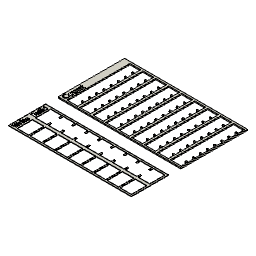
magnetic math (Autodesk Fusion 360 design; units mm, degrees)
Autodesk Fusion 360 part; units mm, degrees
sketch "Sketch3" plane through (0, 0, 0) normal (0, 0, 1) x (1, 0, 0)
  line L0 (672.1477, -0.2754) -> (0.2647, -0.2754)
  line L1 (0.2647, -0.2754) -> (0.2647, -203.3998)
  line L2 (0.2647, -203.3998) -> (672.1477, -203.3998)
  line L3 (672.1477, -203.3998) -> (672.1477, -0.2754)
  line L4 (100.5154, -109.9886) -> (37.7823, -109.9886)
  line L5 (37.7823, -109.9886) -> (37.7823, -193.6499)
  line L6 (37.7823, -193.6499) -> (100.5154, -193.6499)
  line L7 (100.5154, -193.6499) -> (100.5154, -109.9886)
  line L8 (170.7886, -109.9886) -> (108.056, -109.9886)
  line L9 (108.056, -109.9886) -> (108.056, -193.6499)
  line L10 (108.056, -193.6499) -> (170.7886, -193.6499)
  line L11 (170.7886, -193.6499) -> (170.7886, -109.9886)
  line L12 (241.0619, -109.9886) -> (178.3293, -109.9886)
  line L13 (178.3293, -109.9886) -> (178.3293, -193.6499)
  line L14 (178.3293, -193.6499) -> (241.0619, -193.6499)
  line L15 (241.0619, -193.6499) -> (241.0619, -109.9886)
  line L16 (311.3615, -109.9886) -> (248.6025, -109.9886)
  line L17 (248.6025, -109.9886) -> (248.6025, -193.6499)
  line L18 (248.6025, -193.6499) -> (311.3615, -193.6499)
  line L19 (311.3615, -193.6499) -> (311.3615, -109.9886)
  line L20 (381.6352, -109.9886) -> (318.8757, -109.9886)
  line L21 (318.8757, -109.9886) -> (318.8757, -193.6499)
  line L22 (318.8757, -193.6499) -> (381.6352, -193.6499)
  line L23 (381.6352, -193.6499) -> (381.6352, -109.9886)
  line L24 (451.9084, -109.9886) -> (389.149, -109.9886)
  line L25 (389.149, -109.9886) -> (389.149, -193.6499)
  line L26 (389.149, -193.6499) -> (451.9084, -193.6499)
  line L27 (451.9084, -193.6499) -> (451.9084, -109.9886)
  line L28 (522.1817, -109.9886) -> (459.4491, -109.9886)
  line L29 (459.4491, -109.9886) -> (459.4491, -193.6499)
  line L30 (459.4491, -193.6499) -> (522.1817, -193.6499)
  line L31 (522.1817, -193.6499) -> (522.1817, -109.9886)
  line L32 (592.4549, -109.9886) -> (529.7223, -109.9886)
  line L33 (529.7223, -109.9886) -> (529.7223, -193.6499)
  line L34 (529.7223, -193.6499) -> (592.4549, -193.6499)
  line L35 (592.4549, -193.6499) -> (592.4549, -109.9886)
  line L36 (662.7281, -109.9886) -> (599.9955, -109.9886)
  line L37 (599.9955, -109.9886) -> (599.9955, -193.6499)
  line L38 (599.9955, -193.6499) -> (662.7281, -193.6499)
  line L39 (662.7281, -193.6499) -> (662.7281, -109.9886)
  line L40 (100.5154, -28.7041) -> (100.5154, -10.038)
  line L41 (100.5154, -10.038) -> (37.7823, -10.038)
  line L42 (37.7823, -10.038) -> (37.7823, -93.6982)
  line L43 (37.7823, -93.6982) -> (100.5154, -93.6982)
  line L44 (100.5154, -93.6982) -> (100.5154, -75.5793)
  line L45 (100.5154, -75.5793) -> (108.056, -75.5793)
  line L46 (108.056, -75.5793) -> (108.056, -93.6982)
  line L47 (108.056, -93.6982) -> (170.7886, -93.6982)
  line L48 (170.7886, -93.6982) -> (170.7886, -75.5793)
  line L49 (170.7886, -75.5793) -> (178.3293, -75.5793)
  line L50 (178.3293, -75.5793) -> (178.3293, -93.6982)
  line L51 (178.3293, -93.6982) -> (241.0619, -93.6982)
  line L52 (241.0619, -93.6982) -> (241.0619, -75.5793)
  line L53 (241.0619, -75.5793) -> (248.6025, -75.5793)
  line L54 (248.6025, -75.5793) -> (248.6025, -93.6982)
  line L55 (248.6025, -93.6982) -> (311.3615, -93.6982)
  line L56 (311.3615, -93.6982) -> (311.3615, -75.5793)
  line L57 (311.3615, -75.5793) -> (318.8757, -75.5793)
  line L58 (318.8757, -75.5793) -> (318.8757, -93.6982)
  line L59 (318.8757, -93.6982) -> (381.6352, -93.6982)
  line L60 (381.6352, -93.6982) -> (381.6352, -75.5793)
  line L61 (381.6352, -75.5793) -> (389.149, -75.5793)
  line L62 (389.149, -75.5793) -> (389.149, -93.6982)
  line L63 (389.149, -93.6982) -> (451.9084, -93.6982)
  line L64 (451.9084, -93.6982) -> (451.9084, -75.5793)
  line L65 (451.9084, -75.5793) -> (459.4491, -75.5793)
  line L66 (459.4491, -75.5793) -> (459.4491, -93.6982)
  line L67 (459.4491, -93.6982) -> (522.1817, -93.6982)
  line L68 (522.1817, -93.6982) -> (522.1817, -75.5793)
  line L69 (522.1817, -75.5793) -> (529.7223, -75.5793)
  line L70 (529.7223, -75.5793) -> (529.7223, -93.6982)
  line L71 (529.7223, -93.6982) -> (592.4549, -93.6982)
  line L72 (592.4549, -93.6982) -> (592.4549, -75.5793)
  line L73 (592.4549, -75.5793) -> (599.9955, -75.5793)
  line L74 (599.9955, -75.5793) -> (599.9955, -93.6982)
  line L75 (599.9955, -93.6982) -> (662.7281, -93.6982)
  line L76 (662.7281, -93.6982) -> (662.7281, -10.038)
  line L77 (662.7281, -10.038) -> (599.9955, -10.038)
  line L78 (599.9955, -10.038) -> (599.9955, -28.7041)
  line L79 (599.9955, -28.7041) -> (592.4549, -28.7041)
  line L80 (592.4549, -28.7041) -> (592.4549, -10.038)
  line L81 (592.4549, -10.038) -> (529.7223, -10.038)
  line L82 (529.7223, -10.038) -> (529.7223, -28.7041)
  line L83 (529.7223, -28.7041) -> (522.1817, -28.7041)
  line L84 (522.1817, -28.7041) -> (522.1817, -10.038)
  line L85 (522.1817, -10.038) -> (459.4491, -10.038)
  line L86 (459.4491, -10.038) -> (459.4491, -28.7041)
  line L87 (459.4491, -28.7041) -> (451.9084, -28.7041)
  line L88 (451.9084, -28.7041) -> (451.9084, -10.038)
  line L89 (451.9084, -10.038) -> (389.149, -10.038)
  line L90 (389.149, -10.038) -> (389.149, -28.7041)
  line L91 (389.149, -28.7041) -> (381.6352, -28.7041)
  line L92 (381.6352, -28.7041) -> (381.6352, -10.038)
  line L93 (381.6352, -10.038) -> (318.8757, -10.038)
  line L94 (318.8757, -10.038) -> (318.8757, -28.7041)
  line L95 (318.8757, -28.7041) -> (311.3615, -28.7041)
  line L96 (311.3615, -28.7041) -> (311.3615, -10.038)
  line L97 (311.3615, -10.038) -> (248.6025, -10.038)
  line L98 (248.6025, -10.038) -> (248.6025, -28.7041)
  line L99 (248.6025, -28.7041) -> (241.0619, -28.7041)
  line L100 (241.0619, -28.7041) -> (241.0619, -10.038)
  line L101 (241.0619, -10.038) -> (178.3293, -10.038)
  line L102 (178.3293, -10.038) -> (178.3293, -28.7041)
  line L103 (178.3293, -28.7041) -> (170.7886, -28.7041)
  line L104 (170.7886, -28.7041) -> (170.7886, -10.038)
  line L105 (170.7886, -10.038) -> (108.056, -10.038)
  line L106 (108.056, -10.038) -> (108.056, -28.7041)
  line L107 (108.056, -28.7041) -> (100.5154, -28.7041)
  line L108 (28.8958, -89.0962) -> (7.0937, -89.0962)
  line L109 (7.0937, -89.0962) -> (7.0937, -81.6748)
  spline S0 degree 3 poles (7.0937, -81.6748) (7.0937, -79.4876) (7.5059, -77.821) (8.3302, -76.6751) knots 0 0 0 0 1 1 1 1
  spline S1 degree 3 poles (8.3302, -76.6751) (9.1562, -75.5295) (10.3585, -74.9695) (11.9405, -74.9695) knots 0 0 0 0 1 1 1 1
  spline S2 degree 3 poles (11.9405, -74.9695) (14.5623, -74.9695) (16.4179, -76.7013) (17.5091, -80.1905) knots 0 0 0 0 1 1 1 1
  spline S3 degree 3 poles (17.5091, -80.1905) (18.501, -76.1154) (20.4986, -74.0843) (23.5034, -74.0843) knots 0 0 0 0 1 1 1 1
  spline S4 degree 3 poles (23.5034, -74.0843) (25.2428, -74.0843) (26.575, -74.6702) (27.5037, -75.868) knots 0 0 0 0 1 1 1 1
  spline S5 degree 3 poles (27.5037, -75.868) (28.4324, -77.0657) (28.8958, -78.7715) (28.8958, -80.9979) knots 0 0 0 0 1 1 1 1
  line L110 (28.8958, -80.9979) -> (28.8958, -89.0962)
  line L111 (16.1682, -84.8126) -> (16.1682, -83.7451)
  spline S6 degree 3 poles (16.1682, -83.7451) (16.1682, -82.469) (15.8535, -81.4536) (15.2259, -80.6983) knots 0 0 0 0 1 1 1 1
  spline S7 degree 3 poles (15.2259, -80.6983) (14.5965, -79.9563) (13.7414, -79.5787) (12.6622, -79.5787) knots 0 0 0 0 1 1 1 1
  spline S8 degree 3 poles (12.6622, -79.5787) (11.66, -79.5787) (10.9793, -79.8782) (10.6219, -80.4771) knots 0 0 0 0 1 1 1 1
  spline S9 degree 3 poles (10.6219, -80.4771) (10.2628, -81.0889) (10.0832, -82.2218) (10.0832, -83.9012) knots 0 0 0 0 1 1 1 1
  line L112 (10.0832, -83.9012) -> (10.0832, -84.8126)
  line L113 (10.0832, -84.8126) -> (16.1682, -84.8126)
  line L114 (25.802, -84.8126) -> (25.802, -83.8493)
  spline S10 degree 3 poles (25.802, -83.8493) (25.802, -81.9352) (25.5985, -80.6332) (25.1914, -79.9042) knots 0 0 0 0 1 1 1 1
  spline S11 degree 3 poles (25.1914, -79.9042) (24.7827, -79.1881) (24.0405, -78.8234) (22.9596, -78.8234) knots 0 0 0 0 1 1 1 1
  spline S12 degree 3 poles (22.9596, -78.8234) (21.8496, -78.8234) (20.9261, -79.3053) (20.189, -80.2688) knots 0 0 0 0 1 1 1 1
  spline S13 degree 3 poles (20.189, -80.2688) (19.4536, -81.2453) (19.0842, -82.456) (19.0842, -83.9404) knots 0 0 0 0 1 1 1 1
  line L115 (19.0842, -83.9404) -> (19.0842, -84.8126)
  line L116 (19.0842, -84.8126) -> (25.802, -84.8126)
  line L117 (28.8958, -60.0879) -> (25.8465, -60.0879)
  spline S14 degree 3 poles (25.8465, -60.0879) (28.1245, -61.4939) (29.2635, -63.3296) (29.2635, -65.5952) knots 0 0 0 0 1 1 1 1
  spline S15 degree 3 poles (29.2635, -65.5952) (29.2635, -67.0403) (28.8086, -68.1732) (27.8936, -69.0065) knots 0 0 0 0 1 1 1 1
  spline S16 degree 3 poles (27.8936, -69.0065) (26.9804, -69.8528) (25.7336, -70.2694) (24.1533, -70.2694) knots 0 0 0 0 1 1 1 1
  line L118 (24.1533, -70.2694) -> (12.7204, -70.2694)
  line L119 (12.7204, -70.2694) -> (12.7204, -65.9077)
  line L120 (12.7204, -65.9077) -> (23.0776, -65.9077)
  spline S17 degree 3 poles (23.0776, -65.9077) (24.9144, -65.9077) (25.8328, -65.2958) (25.8328, -64.0589) knots 0 0 0 0 1 1 1 1
  spline S18 degree 3 poles (25.8328, -64.0589) (25.8328, -62.6918) (24.8545, -61.3637) (22.8997, -60.0879) knots 0 0 0 0 1 1 1 1
  line L121 (22.8997, -60.0879) -> (12.7204, -60.0879)
  line L122 (12.7204, -60.0879) -> (12.7204, -55.7262)
  line L123 (12.7204, -55.7262) -> (28.8958, -55.7262)
  line L124 (28.8958, -55.7262) -> (28.8958, -60.0879)
  line L125 (28.8958, -50.2707) -> (12.7204, -50.2707)
  line L126 (12.7204, -50.2707) -> (12.7204, -45.909)
  line L127 (12.7204, -45.909) -> (28.8958, -45.909)
  line L128 (28.8958, -45.909) -> (28.8958, -50.2707)
  line L129 (9.996, -50.2707) -> (6.3566, -50.2707)
  line L130 (6.3566, -50.2707) -> (6.3566, -45.909)
  line L131 (6.3566, -45.909) -> (9.996, -45.909)
  line L132 (9.996, -45.909) -> (9.996, -50.2707)
  line L133 (5.6349, -40.4666) -> (5.6349, -36.106)
  line L134 (5.6349, -36.106) -> (28.8965, -36.106)
  line L135 (28.8965, -36.106) -> (28.8965, -40.4666)
  line L136 (28.8965, -40.4666) -> (5.6349, -40.4666)
  line L137 (28.8958, -20.4679) -> (25.8465, -20.4679)
  spline S19 degree 3 poles (25.8465, -20.4679) (28.1245, -21.5876) (29.2635, -23.3583) (29.2635, -25.754) knots 0 0 0 0 1 1 1 1
  spline S20 degree 3 poles (29.2635, -25.754) (29.2635, -27.707) (28.5521, -29.2305) (27.1274, -30.3372) knots 0 0 0 0 1 1 1 1
  spline S21 degree 3 poles (27.1274, -30.3372) (25.7045, -31.4568) (23.7446, -32.0036) (21.2511, -32.0036) knots 0 0 0 0 1 1 1 1
  spline S22 degree 3 poles (21.2511, -32.0036) (18.5403, -32.0036) (16.3786, -31.3788) (14.7675, -30.1287) knots 0 0 0 0 1 1 1 1
  spline S23 degree 3 poles (14.7675, -30.1287) (13.1582, -28.8788) (12.3527, -27.1992) (12.3527, -25.0771) knots 0 0 0 0 1 1 1 1
  spline S24 degree 3 poles (12.3527, -25.0771) (12.3527, -23.3974) (13.0197, -21.861) (14.3554, -20.4679) knots 0 0 0 0 1 1 1 1
  line L138 (14.3554, -20.4679) -> (5.6348, -20.4679)
  line L139 (5.6348, -20.4679) -> (5.6348, -16.0933)
  line L140 (5.6348, -16.0933) -> (28.8958, -16.0933)
  line L141 (28.8958, -16.0933) -> (28.8958, -20.4679)
  spline S25 degree 3 poles (16.9481, -20.4679) (15.7697, -21.5225) (15.1814, -22.6422) (15.1814, -23.8402) knots 0 0 0 0 1 1 1 1
  spline S26 degree 3 poles (15.1814, -23.8402) (15.1814, -24.9207) (15.6962, -25.767) (16.7275, -26.405) knots 0 0 0 0 1 1 1 1
  spline S27 degree 3 poles (16.7275, -26.405) (17.7587, -27.043) (19.144, -27.3685) (20.8816, -27.3685) knots 0 0 0 0 1 1 1 1
  spline S28 degree 3 poles (20.8816, -27.3685) (24.1927, -27.3685) (25.8465, -26.301) (25.8465, -24.1786) knots 0 0 0 0 1 1 1 1
  spline S29 degree 3 poles (25.8465, -24.1786) (25.8465, -22.8896) (25.017, -21.6527) (23.3564, -20.4679) knots 0 0 0 0 1 1 1 1
  line L142 (23.3564, -20.4679) -> (16.9481, -20.4679)
  line L143 (28.8958, -187.9119) -> (7.0937, -193.3379)
  line L144 (7.0937, -193.3379) -> (7.0937, -189.0572)
  line L145 (7.0937, -189.0572) -> (23.0485, -185.0761)
  line L146 (23.0485, -185.0761) -> (7.0937, -181.3269)
  line L147 (7.0937, -181.3269) -> (7.0937, -177.5369)
  line L148 (7.0937, -177.5369) -> (22.9596, -173.9648)
  line L149 (22.9596, -173.9648) -> (7.0937, -169.7794)
  line L150 (7.0937, -169.7794) -> (7.0937, -166.6437)
  line L151 (7.0937, -166.6437) -> (28.8958, -172.3698)
  line L152 (28.8958, -172.3698) -> (28.8958, -176.6915)
  line L153 (28.8958, -176.6915) -> (13.9432, -180.0591)
  line L154 (13.9432, -180.0591) -> (28.8958, -183.5764)
  line L155 (28.8958, -183.5764) -> (28.8958, -187.9119)
  line L156 (28.8958, -163.6579) -> (12.7204, -163.6579)
  line L157 (12.7204, -163.6579) -> (12.7204, -159.2952)
  line L158 (12.7204, -159.2952) -> (15.7697, -159.2952)
  spline S30 degree 3 poles (15.7697, -159.2952) (13.4917, -158.1635) (12.3527, -156.4458) (12.3527, -154.1417) knots 0 0 0 0 1 1 1 1
  spline S31 degree 3 poles (12.3527, -154.1417) (12.3527, -153.869) (12.3818, -153.5963) (12.4399, -153.3237) knots 0 0 0 0 1 1 1 1
  line L159 (12.4399, -153.3237) -> (16.3307, -153.3237)
  spline S32 degree 3 poles (16.3307, -153.3237) (16.1032, -153.951) (15.9904, -154.5235) (15.9904, -155.0553) knots 0 0 0 0 1 1 1 1
  spline S33 degree 3 poles (15.9904, -155.0553) (15.9904, -156.7866) (16.8694, -158.2045) (18.6275, -159.2952) knots 0 0 0 0 1 1 1 1
  line L160 (18.6275, -159.2952) -> (28.8958, -159.2952)
  line L161 (28.8958, -159.2952) -> (28.8958, -163.6579)
  line L162 (28.8958, -149.9427) -> (12.7204, -149.9427)
  line L163 (12.7204, -149.9427) -> (12.7204, -145.58)
  line L164 (12.7204, -145.58) -> (28.8958, -145.58)
  line L165 (28.8958, -145.58) -> (28.8958, -149.9427)
  line L166 (9.996, -149.9427) -> (6.3566, -149.9427)
  line L167 (6.3566, -149.9427) -> (6.3566, -145.58)
  line L168 (6.3566, -145.58) -> (9.996, -145.58)
  line L169 (9.996, -145.58) -> (9.996, -149.9427)
  spline S34 degree 3 poles (28.8086, -131.7966) (29.113, -132.8327) (29.2635, -133.6507) (29.2635, -134.2506) knots 0 0 0 0 1 1 1 1
  spline S35 degree 3 poles (29.2635, -134.2506) (29.2635, -138.027) (27.4969, -139.9221) (23.9601, -139.9221) knots 0 0 0 0 1 1 1 1
  line L170 (23.9601, -139.9221) -> (15.4465, -139.9221)
  line L171 (15.4465, -139.9221) -> (15.4465, -141.7352)
  line L172 (15.4465, -141.7352) -> (12.7204, -141.7352)
  line L173 (12.7204, -141.7352) -> (12.7204, -139.9221)
  line L174 (12.7204, -139.9221) -> (9.996, -139.9221)
  line L175 (9.996, -139.9221) -> (9.4949, -135.5594)
  line L176 (9.4949, -135.5594) -> (12.7204, -135.5594)
  line L177 (12.7204, -135.5594) -> (12.7204, -132.0964)
  line L178 (12.7204, -132.0964) -> (15.4465, -132.0964)
  line L179 (15.4465, -132.0964) -> (15.4465, -135.5594)
  line L180 (15.4465, -135.5594) -> (23.3872, -135.5594)
  spline S36 degree 3 poles (23.3872, -135.5594) (25.371, -135.5594) (26.363, -134.755) (26.363, -133.1325) knots 0 0 0 0 1 1 1 1
  spline S37 degree 3 poles (26.363, -133.1325) (26.363, -132.7645) (26.2928, -132.3145) (26.156, -131.7966) knots 0 0 0 0 1 1 1 1
  line L181 (26.156, -131.7966) -> (28.8086, -131.7966)
  spline S38 degree 3 poles (28.352, -114.7273) (28.9608, -116.7998) (29.2635, -118.7628) (29.2635, -120.6307) knots 0 0 0 0 1 1 1 1
  spline S39 degree 3 poles (29.2635, -120.6307) (29.2635, -123.33) (28.4991, -125.457) (26.9667, -127.0249) knots 0 0 0 0 1 1 1 1
  spline S40 degree 3 poles (26.9667, -127.0249) (25.4343, -128.5789) (23.3427, -129.3562) (20.6901, -129.3562) knots 0 0 0 0 1 1 1 1
  spline S41 degree 3 poles (20.6901, -129.3562) (18.1863, -129.3562) (16.1699, -128.6471) (14.6427, -127.2156) knots 0 0 0 0 1 1 1 1
  spline S42 degree 3 poles (14.6427, -127.2156) (13.1154, -125.784) (12.3527, -123.9028) (12.3527, -121.5577) knots 0 0 0 0 1 1 1 1
  spline S43 degree 3 poles (12.3527, -121.5577) (12.3527, -119.1856) (13.0983, -117.454) (14.5914, -116.3634) knots 0 0 0 0 1 1 1 1
  spline S44 degree 3 poles (14.5914, -116.3634) (16.0844, -115.2727) (18.4463, -114.7273) (21.6769, -114.7273) knots 0 0 0 0 1 1 1 1
  line L182 (21.6769, -114.7273) -> (21.6769, -124.7615)
  spline S45 degree 3 poles (21.6769, -124.7615) (24.7622, -124.4753) (26.3031, -122.7711) (26.3031, -119.6764) knots 0 0 0 0 1 1 1 1
  spline S46 degree 3 poles (26.3031, -119.6764) (26.3031, -118.2175) (25.9645, -116.5679) (25.2872, -114.7273) knots 0 0 0 0 1 1 1 1
  line L183 (25.2872, -114.7273) -> (28.352, -114.7273)
  line L184 (19.2176, -124.8297) -> (19.2176, -119.0219)
  spline S47 degree 3 poles (19.2176, -119.0219) (16.4573, -119.0219) (15.0771, -119.9081) (15.0771, -121.6804) knots 0 0 0 0 1 1 1 1
  spline S48 degree 3 poles (15.0771, -121.6804) (15.0771, -123.4938) (16.4573, -124.5434) (19.2176, -124.8297) knots 0 0 0 0 1 1 1 1
extrude "Extrude3" add sketch "Sketch3" along normal blind 2 contours L0 L1 L2 L3 makes body 1
scale "Scale3" factor 0.32 about (0.2647, -203.3998, 2) bodies 1
sketch "Sketch5" plane through (0, 0, 0) normal (0, 0, 1) x (1, 0, 0)
  line L0 (215.0872, -0.0882) -> (0.0847, -0.0882)
  line L1 (0.0847, -0.0882) -> (0.0847, -116.5435)
  line L2 (0.0847, -116.5435) -> (215.0872, -116.5435)
  line L3 (215.0872, -116.5435) -> (215.0872, -0.0882)
  line L4 (27.5336, -13.7736) -> (31.5892, -13.7736)
  line L5 (31.5892, -13.7736) -> (31.5892, -3.2736)
  line L6 (31.5892, -3.2736) -> (12.5899, -3.2736)
  line L7 (12.5899, -3.2736) -> (12.5899, -7.2379)
  line L8 (12.5899, -7.2379) -> (12.5307, -7.2379)
  line L9 (12.5307, -7.2379) -> (12.5307, -109.3934)
  line L10 (12.5307, -109.3934) -> (12.5899, -109.3934)
  line L11 (12.5899, -109.3934) -> (12.5899, -113.7732)
  line L12 (12.5899, -113.7732) -> (31.5892, -113.7732)
  line L13 (31.5892, -113.7732) -> (31.5892, -103.2737)
  line L14 (31.5892, -103.2737) -> (27.5336, -103.2737)
  line L15 (27.5336, -103.2737) -> (27.5336, -101.2739)
  line L16 (27.5336, -101.2739) -> (31.5892, -101.2739)
  line L17 (31.5892, -101.2739) -> (31.5892, -90.7735)
  line L18 (31.5892, -90.7735) -> (27.5336, -90.7735)
  line L19 (27.5336, -90.7735) -> (27.5336, -88.7737)
  line L20 (27.5336, -88.7737) -> (31.5892, -88.7737)
  line L21 (31.5892, -88.7737) -> (31.5892, -78.2733)
  line L22 (31.5892, -78.2733) -> (27.5336, -78.2733)
  line L23 (27.5336, -78.2733) -> (27.5336, -76.2735)
  line L24 (27.5336, -76.2735) -> (31.5892, -76.2735)
  line L25 (31.5892, -76.2735) -> (31.5892, -65.774)
  line L26 (31.5892, -65.774) -> (27.5336, -65.774)
  line L27 (27.5336, -65.774) -> (27.5336, -63.7733)
  line L28 (27.5336, -63.7733) -> (31.5892, -63.7733)
  line L29 (31.5892, -63.7733) -> (31.5892, -53.2738)
  line L30 (31.5892, -53.2738) -> (27.5336, -53.2738)
  line L31 (27.5336, -53.2738) -> (27.5336, -51.274)
  line L32 (27.5336, -51.274) -> (31.5892, -51.274)
  line L33 (31.5892, -51.274) -> (31.5892, -40.7736)
  line L34 (31.5892, -40.7736) -> (27.5336, -40.7736)
  line L35 (27.5336, -40.7736) -> (27.5336, -38.7738)
  line L36 (27.5336, -38.7738) -> (31.5892, -38.7738)
  line L37 (31.5892, -38.7738) -> (31.5892, -28.2734)
  line L38 (31.5892, -28.2734) -> (27.5336, -28.2734)
  line L39 (27.5336, -28.2734) -> (27.5336, -26.2735)
  line L40 (27.5336, -26.2735) -> (31.5892, -26.2735)
  line L41 (31.5892, -26.2735) -> (31.5892, -15.7736)
  line L42 (31.5892, -15.7736) -> (27.5336, -15.7736)
  line L43 (27.5336, -15.7736) -> (27.5336, -13.7736)
  line L44 (50.2073, -13.7736) -> (54.2713, -13.7736)
  line L45 (54.2713, -13.7736) -> (54.2713, -3.2736)
  line L46 (54.2713, -3.2736) -> (35.2722, -3.2736)
  line L47 (35.2722, -3.2736) -> (35.2722, -7.2379)
  line L48 (35.2722, -7.2379) -> (35.2044, -7.2379)
  line L49 (35.2044, -7.2379) -> (35.2044, -109.3934)
  line L50 (35.2044, -109.3934) -> (35.2722, -109.3934)
  line L51 (35.2722, -109.3934) -> (35.2722, -113.7732)
  line L52 (35.2722, -113.7732) -> (54.2713, -113.7732)
  line L53 (54.2713, -113.7732) -> (54.2713, -103.2737)
  line L54 (54.2713, -103.2737) -> (50.2073, -103.2737)
  line L55 (50.2073, -103.2737) -> (50.2073, -101.2739)
  line L56 (50.2073, -101.2739) -> (54.2713, -101.2739)
  line L57 (54.2713, -101.2739) -> (54.2713, -90.7735)
  line L58 (54.2713, -90.7735) -> (50.2073, -90.7735)
  line L59 (50.2073, -90.7735) -> (50.2073, -88.7737)
  line L60 (50.2073, -88.7737) -> (54.2713, -88.7737)
  line L61 (54.2713, -88.7737) -> (54.2713, -78.2733)
  line L62 (54.2713, -78.2733) -> (50.2073, -78.2733)
  line L63 (50.2073, -78.2733) -> (50.2073, -76.2735)
  line L64 (50.2073, -76.2735) -> (54.2713, -76.2735)
  line L65 (54.2713, -76.2735) -> (54.2713, -65.774)
  line L66 (54.2713, -65.774) -> (50.2073, -65.774)
  line L67 (50.2073, -65.774) -> (50.2073, -63.7733)
  line L68 (50.2073, -63.7733) -> (54.2713, -63.7733)
  line L69 (54.2713, -63.7733) -> (54.2713, -53.2738)
  line L70 (54.2713, -53.2738) -> (50.2073, -53.2738)
  line L71 (50.2073, -53.2738) -> (50.2073, -51.274)
  line L72 (50.2073, -51.274) -> (54.2713, -51.274)
  line L73 (54.2713, -51.274) -> (54.2713, -40.7736)
  line L74 (54.2713, -40.7736) -> (50.2073, -40.7736)
  line L75 (50.2073, -40.7736) -> (50.2073, -38.7738)
  line L76 (50.2073, -38.7738) -> (54.2713, -38.7738)
  line L77 (54.2713, -38.7738) -> (54.2713, -28.2734)
  line L78 (54.2713, -28.2734) -> (50.2073, -28.2734)
  line L79 (50.2073, -28.2734) -> (50.2073, -26.2735)
  line L80 (50.2073, -26.2735) -> (54.2713, -26.2735)
  line L81 (54.2713, -26.2735) -> (54.2713, -15.7736)
  line L82 (54.2713, -15.7736) -> (50.2073, -15.7736)
  line L83 (50.2073, -15.7736) -> (50.2073, -13.7736)
  line L84 (72.881, -13.7736) -> (76.945, -13.7736)
  line L85 (76.945, -13.7736) -> (76.945, -3.2736)
  line L86 (76.945, -3.2736) -> (57.9459, -3.2736)
  line L87 (57.9459, -3.2736) -> (57.9459, -7.2379)
  line L88 (57.9459, -7.2379) -> (57.8782, -7.2379)
  line L89 (57.8782, -7.2379) -> (57.8782, -109.3934)
  line L90 (57.8782, -109.3934) -> (57.9459, -109.3934)
  line L91 (57.9459, -109.3934) -> (57.9459, -113.7732)
  line L92 (57.9459, -113.7732) -> (76.945, -113.7732)
  line L93 (76.945, -113.7732) -> (76.945, -103.2737)
  line L94 (76.945, -103.2737) -> (72.881, -103.2737)
  line L95 (72.881, -103.2737) -> (72.881, -101.2739)
  line L96 (72.881, -101.2739) -> (76.945, -101.2739)
  line L97 (76.945, -101.2739) -> (76.945, -90.7735)
  line L98 (76.945, -90.7735) -> (72.881, -90.7735)
  line L99 (72.881, -90.7735) -> (72.881, -88.7737)
  line L100 (72.881, -88.7737) -> (76.945, -88.7737)
  line L101 (76.945, -88.7737) -> (76.945, -78.2733)
  line L102 (76.945, -78.2733) -> (72.881, -78.2733)
  line L103 (72.881, -78.2733) -> (72.881, -76.2735)
  line L104 (72.881, -76.2735) -> (76.945, -76.2735)
  line L105 (76.945, -76.2735) -> (76.945, -65.774)
  line L106 (76.945, -65.774) -> (72.881, -65.774)
  line L107 (72.881, -65.774) -> (72.881, -63.7733)
  line L108 (72.881, -63.7733) -> (76.945, -63.7733)
  line L109 (76.945, -63.7733) -> (76.945, -53.2738)
  line L110 (76.945, -53.2738) -> (72.881, -53.2738)
  line L111 (72.881, -53.2738) -> (72.881, -51.274)
  line L112 (72.881, -51.274) -> (76.945, -51.274)
  line L113 (76.945, -51.274) -> (76.945, -40.7736)
  line L114 (76.945, -40.7736) -> (72.881, -40.7736)
  line L115 (72.881, -40.7736) -> (72.881, -38.7738)
  line L116 (72.881, -38.7738) -> (76.945, -38.7738)
  line L117 (76.945, -38.7738) -> (76.945, -28.2734)
  line L118 (76.945, -28.2734) -> (72.881, -28.2734)
  line L119 (72.881, -28.2734) -> (72.881, -26.2735)
  line L120 (72.881, -26.2735) -> (76.945, -26.2735)
  line L121 (76.945, -26.2735) -> (76.945, -15.7736)
  line L122 (76.945, -15.7736) -> (72.881, -15.7736)
  line L123 (72.881, -15.7736) -> (72.881, -13.7736)
  line L124 (95.5548, -13.7736) -> (99.6188, -13.7736)
  line L125 (99.6188, -13.7736) -> (99.6188, -3.2736)
  line L126 (99.6188, -3.2736) -> (80.6196, -3.2736)
  line L127 (80.6196, -3.2736) -> (80.6196, -7.2379)
  line L128 (80.6196, -7.2379) -> (80.5519, -7.2379)
  line L129 (80.5519, -7.2379) -> (80.5519, -109.3934)
  line L130 (80.5519, -109.3934) -> (80.6196, -109.3934)
  line L131 (80.6196, -109.3934) -> (80.6196, -113.7732)
  line L132 (80.6196, -113.7732) -> (99.6188, -113.7732)
  line L133 (99.6188, -113.7732) -> (99.6188, -103.2737)
  line L134 (99.6188, -103.2737) -> (95.5548, -103.2737)
  line L135 (95.5548, -103.2737) -> (95.5548, -101.2739)
  line L136 (95.5548, -101.2739) -> (99.6188, -101.2739)
  line L137 (99.6188, -101.2739) -> (99.6188, -90.7735)
  line L138 (99.6188, -90.7735) -> (95.5548, -90.7735)
  line L139 (95.5548, -90.7735) -> (95.5548, -88.7737)
  line L140 (95.5548, -88.7737) -> (99.6188, -88.7737)
  line L141 (99.6188, -88.7737) -> (99.6188, -78.2733)
  line L142 (99.6188, -78.2733) -> (95.5548, -78.2733)
  line L143 (95.5548, -78.2733) -> (95.5548, -76.2735)
  line L144 (95.5548, -76.2735) -> (99.6188, -76.2735)
  line L145 (99.6188, -76.2735) -> (99.6188, -65.774)
  line L146 (99.6188, -65.774) -> (95.5548, -65.774)
  line L147 (95.5548, -65.774) -> (95.5548, -63.7733)
  line L148 (95.5548, -63.7733) -> (99.6188, -63.7733)
  line L149 (99.6188, -63.7733) -> (99.6188, -53.2738)
  line L150 (99.6188, -53.2738) -> (95.5548, -53.2738)
  line L151 (95.5548, -53.2738) -> (95.5548, -51.274)
  line L152 (95.5548, -51.274) -> (99.6188, -51.274)
  line L153 (99.6188, -51.274) -> (99.6188, -40.7736)
  line L154 (99.6188, -40.7736) -> (95.5548, -40.7736)
  line L155 (95.5548, -40.7736) -> (95.5548, -38.7738)
  line L156 (95.5548, -38.7738) -> (99.6188, -38.7738)
  line L157 (99.6188, -38.7738) -> (99.6188, -28.2734)
  line L158 (99.6188, -28.2734) -> (95.5548, -28.2734)
  line L159 (95.5548, -28.2734) -> (95.5548, -26.2735)
  line L160 (95.5548, -26.2735) -> (99.6188, -26.2735)
  line L161 (99.6188, -26.2735) -> (99.6188, -15.7736)
  line L162 (99.6188, -15.7736) -> (95.5548, -15.7736)
  line L163 (95.5548, -15.7736) -> (95.5548, -13.7736)
  line L164 (118.2285, -13.7736) -> (122.2925, -13.7736)
  line L165 (122.2925, -13.7736) -> (122.2925, -3.2736)
  line L166 (122.2925, -3.2736) -> (103.2933, -3.2736)
  line L167 (103.2933, -3.2736) -> (103.2933, -7.2379)
  line L168 (103.2933, -7.2379) -> (103.2256, -7.2379)
  line L169 (103.2256, -7.2379) -> (103.2256, -109.3934)
  line L170 (103.2256, -109.3934) -> (103.2933, -109.3934)
  line L171 (103.2933, -109.3934) -> (103.2933, -113.7732)
  line L172 (103.2933, -113.7732) -> (122.2925, -113.7732)
  line L173 (122.2925, -113.7732) -> (122.2925, -103.2737)
  line L174 (122.2925, -103.2737) -> (118.2285, -103.2737)
  line L175 (118.2285, -103.2737) -> (118.2285, -101.2739)
  line L176 (118.2285, -101.2739) -> (122.2925, -101.2739)
  line L177 (122.2925, -101.2739) -> (122.2925, -90.7735)
  line L178 (122.2925, -90.7735) -> (118.2285, -90.7735)
  line L179 (118.2285, -90.7735) -> (118.2285, -88.7737)
  line L180 (118.2285, -88.7737) -> (122.2925, -88.7737)
  line L181 (122.2925, -88.7737) -> (122.2925, -78.2733)
  line L182 (122.2925, -78.2733) -> (118.2285, -78.2733)
  line L183 (118.2285, -78.2733) -> (118.2285, -76.2735)
  line L184 (118.2285, -76.2735) -> (122.2925, -76.2735)
  line L185 (122.2925, -76.2735) -> (122.2925, -65.774)
  line L186 (122.2925, -65.774) -> (118.2285, -65.774)
  line L187 (118.2285, -65.774) -> (118.2285, -63.7733)
  line L188 (118.2285, -63.7733) -> (122.2925, -63.7733)
  line L189 (122.2925, -63.7733) -> (122.2925, -53.2738)
  line L190 (122.2925, -53.2738) -> (118.2285, -53.2738)
  line L191 (118.2285, -53.2738) -> (118.2285, -51.274)
  line L192 (118.2285, -51.274) -> (122.2925, -51.274)
  line L193 (122.2925, -51.274) -> (122.2925, -40.7736)
  line L194 (122.2925, -40.7736) -> (118.2285, -40.7736)
  line L195 (118.2285, -40.7736) -> (118.2285, -38.7738)
  line L196 (118.2285, -38.7738) -> (122.2925, -38.7738)
  line L197 (122.2925, -38.7738) -> (122.2925, -28.2734)
  line L198 (122.2925, -28.2734) -> (118.2285, -28.2734)
  line L199 (118.2285, -28.2734) -> (118.2285, -26.2735)
  line L200 (118.2285, -26.2735) -> (122.2925, -26.2735)
  line L201 (122.2925, -26.2735) -> (122.2925, -15.7736)
  line L202 (122.2925, -15.7736) -> (118.2285, -15.7736)
  line L203 (118.2285, -15.7736) -> (118.2285, -13.7736)
  line L204 (140.9023, -13.7736) -> (144.9747, -13.7736)
  line L205 (144.9747, -13.7736) -> (144.9747, -3.2736)
  line L206 (144.9747, -3.2736) -> (125.967, -3.2736)
  line L207 (125.967, -3.2736) -> (125.967, -7.2379)
  line L208 (125.967, -7.2379) -> (125.8993, -7.2379)
  line L209 (125.8993, -7.2379) -> (125.8993, -109.3934)
  line L210 (125.8993, -109.3934) -> (125.967, -109.3934)
  line L211 (125.967, -109.3934) -> (125.967, -113.7732)
  line L212 (125.967, -113.7732) -> (144.9747, -113.7732)
  line L213 (144.9747, -113.7732) -> (144.9747, -103.2737)
  line L214 (144.9747, -103.2737) -> (140.9023, -103.2737)
  line L215 (140.9023, -103.2737) -> (140.9023, -101.2739)
  line L216 (140.9023, -101.2739) -> (144.9747, -101.2739)
  line L217 (144.9747, -101.2739) -> (144.9747, -90.7735)
  line L218 (144.9747, -90.7735) -> (140.9023, -90.7735)
  line L219 (140.9023, -90.7735) -> (140.9023, -88.7737)
  line L220 (140.9023, -88.7737) -> (144.9747, -88.7737)
  line L221 (144.9747, -88.7737) -> (144.9747, -78.2733)
  line L222 (144.9747, -78.2733) -> (140.9023, -78.2733)
  line L223 (140.9023, -78.2733) -> (140.9023, -76.2735)
  line L224 (140.9023, -76.2735) -> (144.9747, -76.2735)
  line L225 (144.9747, -76.2735) -> (144.9747, -65.774)
  line L226 (144.9747, -65.774) -> (140.9023, -65.774)
  line L227 (140.9023, -65.774) -> (140.9023, -63.7733)
  line L228 (140.9023, -63.7733) -> (144.9747, -63.7733)
  line L229 (144.9747, -63.7733) -> (144.9747, -53.2738)
  line L230 (144.9747, -53.2738) -> (140.9023, -53.2738)
  line L231 (140.9023, -53.2738) -> (140.9023, -51.274)
  line L232 (140.9023, -51.274) -> (144.9747, -51.274)
  line L233 (144.9747, -51.274) -> (144.9747, -40.7736)
  line L234 (144.9747, -40.7736) -> (140.9023, -40.7736)
  line L235 (140.9023, -40.7736) -> (140.9023, -38.7738)
  line L236 (140.9023, -38.7738) -> (144.9747, -38.7738)
  line L237 (144.9747, -38.7738) -> (144.9747, -28.2734)
  line L238 (144.9747, -28.2734) -> (140.9023, -28.2734)
  line L239 (140.9023, -28.2734) -> (140.9023, -26.2735)
  line L240 (140.9023, -26.2735) -> (144.9747, -26.2735)
  line L241 (144.9747, -26.2735) -> (144.9747, -15.7736)
  line L242 (144.9747, -15.7736) -> (140.9023, -15.7736)
  line L243 (140.9023, -15.7736) -> (140.9023, -13.7736)
  line L244 (163.576, -13.7736) -> (167.6485, -13.7736)
  line L245 (167.6485, -13.7736) -> (167.6485, -3.2736)
  line L246 (167.6485, -3.2736) -> (148.6493, -3.2736)
  line L247 (148.6493, -3.2736) -> (148.6493, -7.2379)
  line L248 (148.6493, -7.2379) -> (148.573, -7.2379)
  line L249 (148.573, -7.2379) -> (148.573, -109.3934)
  line L250 (148.573, -109.3934) -> (148.6493, -109.3934)
  line L251 (148.6493, -109.3934) -> (148.6493, -113.7732)
  line L252 (148.6493, -113.7732) -> (167.6485, -113.7732)
  line L253 (167.6485, -113.7732) -> (167.6485, -103.2737)
  line L254 (167.6485, -103.2737) -> (163.576, -103.2737)
  line L255 (163.576, -103.2737) -> (163.576, -101.2739)
  line L256 (163.576, -101.2739) -> (167.6485, -101.2739)
  line L257 (167.6485, -101.2739) -> (167.6485, -90.7735)
  line L258 (167.6485, -90.7735) -> (163.576, -90.7735)
  line L259 (163.576, -90.7735) -> (163.576, -88.7737)
  line L260 (163.576, -88.7737) -> (167.6485, -88.7737)
  line L261 (167.6485, -88.7737) -> (167.6485, -78.2733)
  line L262 (167.6485, -78.2733) -> (163.576, -78.2733)
  line L263 (163.576, -78.2733) -> (163.576, -76.2735)
  line L264 (163.576, -76.2735) -> (167.6485, -76.2735)
  line L265 (167.6485, -76.2735) -> (167.6485, -65.774)
  line L266 (167.6485, -65.774) -> (163.576, -65.774)
  line L267 (163.576, -65.774) -> (163.576, -63.7733)
  line L268 (163.576, -63.7733) -> (167.6485, -63.7733)
  line L269 (167.6485, -63.7733) -> (167.6485, -53.2738)
  line L270 (167.6485, -53.2738) -> (163.576, -53.2738)
  line L271 (163.576, -53.2738) -> (163.576, -51.274)
  line L272 (163.576, -51.274) -> (167.6485, -51.274)
  line L273 (167.6485, -51.274) -> (167.6485, -40.7736)
  line L274 (167.6485, -40.7736) -> (163.576, -40.7736)
  line L275 (163.576, -40.7736) -> (163.576, -38.7738)
  line L276 (163.576, -38.7738) -> (167.6485, -38.7738)
  line L277 (167.6485, -38.7738) -> (167.6485, -28.2734)
  line L278 (167.6485, -28.2734) -> (163.576, -28.2734)
  line L279 (163.576, -28.2734) -> (163.576, -26.2735)
  line L280 (163.576, -26.2735) -> (167.6485, -26.2735)
  line L281 (167.6485, -26.2735) -> (167.6485, -15.7736)
  line L282 (167.6485, -15.7736) -> (163.576, -15.7736)
  line L283 (163.576, -15.7736) -> (163.576, -13.7736)
  line L284 (186.2497, -13.7736) -> (190.3222, -13.7736)
  line L285 (190.3222, -13.7736) -> (190.3222, -3.2736)
  line L286 (190.3222, -3.2736) -> (171.323, -3.2736)
  line L287 (171.323, -3.2736) -> (171.323, -7.2379)
  line L288 (171.323, -7.2379) -> (171.2468, -7.2379)
  line L289 (171.2468, -7.2379) -> (171.2468, -109.3934)
  line L290 (171.2468, -109.3934) -> (171.323, -109.3934)
  line L291 (171.323, -109.3934) -> (171.323, -113.7732)
  line L292 (171.323, -113.7732) -> (190.3222, -113.7732)
  line L293 (190.3222, -113.7732) -> (190.3222, -103.2737)
  line L294 (190.3222, -103.2737) -> (186.2497, -103.2737)
  line L295 (186.2497, -103.2737) -> (186.2497, -101.2739)
  line L296 (186.2497, -101.2739) -> (190.3222, -101.2739)
  line L297 (190.3222, -101.2739) -> (190.3222, -90.7735)
  line L298 (190.3222, -90.7735) -> (186.2497, -90.7735)
  line L299 (186.2497, -90.7735) -> (186.2497, -88.7737)
  line L300 (186.2497, -88.7737) -> (190.3222, -88.7737)
  line L301 (190.3222, -88.7737) -> (190.3222, -78.2733)
  line L302 (190.3222, -78.2733) -> (186.2497, -78.2733)
  line L303 (186.2497, -78.2733) -> (186.2497, -76.2735)
  line L304 (186.2497, -76.2735) -> (190.3222, -76.2735)
  line L305 (190.3222, -76.2735) -> (190.3222, -65.774)
  line L306 (190.3222, -65.774) -> (186.2497, -65.774)
  line L307 (186.2497, -65.774) -> (186.2497, -63.7733)
  line L308 (186.2497, -63.7733) -> (190.3222, -63.7733)
  line L309 (190.3222, -63.7733) -> (190.3222, -53.2738)
  line L310 (190.3222, -53.2738) -> (186.2497, -53.2738)
  line L311 (186.2497, -53.2738) -> (186.2497, -51.274)
  line L312 (186.2497, -51.274) -> (190.3222, -51.274)
  line L313 (190.3222, -51.274) -> (190.3222, -40.7736)
  line L314 (190.3222, -40.7736) -> (186.2497, -40.7736)
  line L315 (186.2497, -40.7736) -> (186.2497, -38.7738)
  line L316 (186.2497, -38.7738) -> (190.3222, -38.7738)
  line L317 (190.3222, -38.7738) -> (190.3222, -28.2734)
  line L318 (190.3222, -28.2734) -> (186.2497, -28.2734)
  line L319 (186.2497, -28.2734) -> (186.2497, -26.2735)
  line L320 (186.2497, -26.2735) -> (190.3222, -26.2735)
  line L321 (190.3222, -26.2735) -> (190.3222, -15.7736)
  line L322 (190.3222, -15.7736) -> (186.2497, -15.7736)
  line L323 (186.2497, -15.7736) -> (186.2497, -13.7736)
  line L324 (208.9235, -13.7736) -> (212.9959, -13.7736)
  line L325 (212.9959, -13.7736) -> (212.9959, -3.2736)
  line L326 (212.9959, -3.2736) -> (193.9967, -3.2736)
  line L327 (193.9967, -3.2736) -> (193.9967, -7.2379)
  line L328 (193.9967, -7.2379) -> (193.9205, -7.2379)
  line L329 (193.9205, -7.2379) -> (193.9205, -109.3934)
  line L330 (193.9205, -109.3934) -> (193.9967, -109.3934)
  line L331 (193.9967, -109.3934) -> (193.9967, -113.7732)
  line L332 (193.9967, -113.7732) -> (212.9959, -113.7732)
  line L333 (212.9959, -113.7732) -> (212.9959, -103.2737)
  line L334 (212.9959, -103.2737) -> (208.9235, -103.2737)
  line L335 (208.9235, -103.2737) -> (208.9235, -101.2739)
  line L336 (208.9235, -101.2739) -> (212.9959, -101.2739)
  line L337 (212.9959, -101.2739) -> (212.9959, -90.7735)
  line L338 (212.9959, -90.7735) -> (208.9235, -90.7735)
  line L339 (208.9235, -90.7735) -> (208.9235, -88.7737)
  line L340 (208.9235, -88.7737) -> (212.9959, -88.7737)
  line L341 (212.9959, -88.7737) -> (212.9959, -78.2733)
  line L342 (212.9959, -78.2733) -> (208.9235, -78.2733)
  line L343 (208.9235, -78.2733) -> (208.9235, -76.2735)
  line L344 (208.9235, -76.2735) -> (212.9959, -76.2735)
  line L345 (212.9959, -76.2735) -> (212.9959, -65.774)
  line L346 (212.9959, -65.774) -> (208.9235, -65.774)
  line L347 (208.9235, -65.774) -> (208.9235, -63.7733)
  line L348 (208.9235, -63.7733) -> (212.9959, -63.7733)
  line L349 (212.9959, -63.7733) -> (212.9959, -53.2738)
  line L350 (212.9959, -53.2738) -> (208.9235, -53.2738)
  line L351 (208.9235, -53.2738) -> (208.9235, -51.274)
  line L352 (208.9235, -51.274) -> (212.9959, -51.274)
  line L353 (212.9959, -51.274) -> (212.9959, -40.7736)
  line L354 (212.9959, -40.7736) -> (208.9235, -40.7736)
  line L355 (208.9235, -40.7736) -> (208.9235, -38.7738)
  line L356 (208.9235, -38.7738) -> (212.9959, -38.7738)
  line L357 (212.9959, -38.7738) -> (212.9959, -28.2734)
  line L358 (212.9959, -28.2734) -> (208.9235, -28.2734)
  line L359 (208.9235, -28.2734) -> (208.9235, -26.2735)
  line L360 (208.9235, -26.2735) -> (212.9959, -26.2735)
  line L361 (212.9959, -26.2735) -> (212.9959, -15.7736)
  line L362 (212.9959, -15.7736) -> (208.9235, -15.7736)
  line L363 (208.9235, -15.7736) -> (208.9235, -13.7736)
  spline S0 degree 3 poles (10.0193, -105.9355) (10.384, -106.7532) (10.5661, -107.7277) (10.5661, -108.8591) knots 0 0 0 0 1 1 1 1
  spline S1 degree 3 poles (10.5661, -108.8591) (10.5661, -110.2408) (10.177, -111.3154) (9.3983, -112.0864) knots 0 0 0 0 1 1 1 1
  spline S2 degree 3 poles (9.3983, -112.0864) (8.6202, -112.8573) (7.534, -113.2445) (6.1407, -113.2445) knots 0 0 0 0 1 1 1 1
  spline S3 degree 3 poles (6.1407, -113.2445) (4.7206, -113.2445) (3.628, -112.854) (2.8631, -112.0797) knots 0 0 0 0 1 1 1 1
  spline S4 degree 3 poles (2.8631, -112.0797) (2.0976, -111.3021) (1.7154, -110.194) (1.7154, -108.7556) knots 0 0 0 0 1 1 1 1
  spline S5 degree 3 poles (1.7154, -108.7556) (1.7154, -107.8378) (1.8237, -106.9234) (2.04, -106.0156) knots 0 0 0 0 1 1 1 1
  line L364 (2.04, -106.0156) -> (3.4128, -106.0156)
  spline S6 degree 3 poles (3.4128, -106.0156) (3.052, -107.0435) (2.8714, -107.9079) (2.8714, -108.6021) knots 0 0 0 0 1 1 1 1
  spline S7 degree 3 poles (2.8714, -108.6021) (2.8714, -109.4899) (3.1535, -110.174) (3.7174, -110.658) knots 0 0 0 0 1 1 1 1
  spline S8 degree 3 poles (3.7174, -110.658) (4.2812, -111.1386) (5.0814, -111.3822) (6.1178, -111.3822) knots 0 0 0 0 1 1 1 1
  spline S9 degree 3 poles (6.1178, -111.3822) (7.1356, -111.3822) (7.9289, -111.1219) (8.4986, -110.6046) knots 0 0 0 0 1 1 1 1
  spline S10 degree 3 poles (8.4986, -110.6046) (9.0683, -110.0839) (9.3529, -109.3664) (9.3529, -108.4419) knots 0 0 0 0 1 1 1 1
  spline S11 degree 3 poles (9.3529, -108.4419) (9.3529, -107.6142) (9.144, -106.7799) (8.7266, -105.9355) knots 0 0 0 0 1 1 1 1
  line L365 (8.7266, -105.9355) -> (10.0193, -105.9355)
  spline S12 degree 3 poles (10.4977, -101.7837) (10.4977, -102.7616) (10.2024, -103.5359) (9.6122, -104.1099) knots 0 0 0 0 1 1 1 1
  spline S13 degree 3 poles (9.6122, -104.1099) (9.0215, -104.6873) (8.2272, -104.9743) (7.2284, -104.9743) knots 0 0 0 0 1 1 1 1
  spline S14 degree 3 poles (7.2284, -104.9743) (6.2183, -104.9743) (5.4211, -104.6839) (4.8363, -104.1066) knots 0 0 0 0 1 1 1 1
  spline S15 degree 3 poles (4.8363, -104.1066) (4.2515, -103.5259) (3.9595, -102.7382) (3.9595, -101.7437) knots 0 0 0 0 1 1 1 1
  spline S16 degree 3 poles (3.9595, -101.7437) (3.9595, -100.7458) (4.2515, -99.9582) (4.8363, -99.3774) knots 0 0 0 0 1 1 1 1
  spline S17 degree 3 poles (4.8363, -99.3774) (5.4211, -98.8001) (6.2149, -98.5097) (7.2171, -98.5097) knots 0 0 0 0 1 1 1 1
  spline S18 degree 3 poles (7.2171, -98.5097) (8.2423, -98.5097) (9.0454, -98.8001) (9.6263, -99.3808) knots 0 0 0 0 1 1 1 1
  spline S19 degree 3 poles (9.6263, -99.3808) (10.2073, -99.9615) (10.4977, -100.7625) (10.4977, -101.7837) knots 0 0 0 0 1 1 1 1
  spline S20 degree 3 poles (9.4442, -101.757) (9.4442, -100.7858) (8.7017, -100.3019) (7.2171, -100.3019) knots 0 0 0 0 1 1 1 1
  spline S21 degree 3 poles (7.2171, -100.3019) (6.5376, -100.3019) (6.0001, -100.432) (5.6052, -100.689) knots 0 0 0 0 1 1 1 1
  spline S22 degree 3 poles (5.6052, -100.689) (5.2102, -100.9427) (5.013, -101.2965) (5.013, -101.7437) knots 0 0 0 0 1 1 1 1
  spline S23 degree 3 poles (5.013, -101.7437) (5.013, -102.1876) (5.2102, -102.538) (5.6052, -102.795) knots 0 0 0 0 1 1 1 1
  spline S24 degree 3 poles (5.6052, -102.795) (6.0001, -103.0519) (6.541, -103.1788) (7.2284, -103.1788) knots 0 0 0 0 1 1 1 1
  spline S25 degree 3 poles (7.2284, -103.1788) (7.9084, -103.1788) (8.4474, -103.0519) (8.8462, -102.7983) knots 0 0 0 0 1 1 1 1
  spline S26 degree 3 poles (8.8462, -102.7983) (9.2446, -102.5447) (9.4442, -102.1976) (9.4442, -101.757) knots 0 0 0 0 1 1 1 1
  line L366 (10.3552, -93.0931) -> (9.1762, -93.0931)
  spline S27 degree 3 poles (9.1762, -93.0931) (10.0574, -93.6404) (10.4977, -94.3513) (10.4977, -95.2223) knots 0 0 0 0 1 1 1 1
  spline S28 degree 3 poles (10.4977, -95.2223) (10.4977, -95.7797) (10.321, -96.2202) (9.9681, -96.5439) knots 0 0 0 0 1 1 1 1
  spline S29 degree 3 poles (9.9681, -96.5439) (9.6151, -96.8677) (9.1328, -97.0279) (8.5216, -97.0279) knots 0 0 0 0 1 1 1 1
  line L367 (8.5216, -97.0279) -> (4.1016, -97.0279)
  line L368 (4.1016, -97.0279) -> (4.1016, -95.3425)
  line L369 (4.1016, -95.3425) -> (8.1056, -95.3425)
  spline S30 degree 3 poles (8.1056, -95.3425) (8.8159, -95.3425) (9.1708, -95.1055) (9.1708, -94.6316) knots 0 0 0 0 1 1 1 1
  spline S31 degree 3 poles (9.1708, -94.6316) (9.1708, -94.0976) (8.793, -93.587) (8.0373, -93.0931) knots 0 0 0 0 1 1 1 1
  line L370 (8.0373, -93.0931) -> (4.1016, -93.0931)
  line L371 (4.1016, -93.0931) -> (4.1016, -91.4076)
  line L372 (4.1016, -91.4076) -> (10.3552, -91.4076)
  line L373 (10.3552, -91.4076) -> (10.3552, -93.0931)
  line L374 (10.3552, -89.2984) -> (4.1016, -89.2984)
  line L375 (4.1016, -89.2984) -> (4.1016, -87.613)
  line L376 (4.1016, -87.613) -> (5.2805, -87.613)
  spline S32 degree 3 poles (5.2805, -87.613) (4.3999, -87.0623) (3.9595, -86.3548) (3.9595, -85.4837) knots 0 0 0 0 1 1 1 1
  spline S33 degree 3 poles (3.9595, -85.4837) (3.9595, -84.9263) (4.1357, -84.4858) (4.4892, -84.1621) knots 0 0 0 0 1 1 1 1
  spline S34 degree 3 poles (4.4892, -84.1621) (4.8422, -83.8384) (5.3245, -83.6781) (5.9357, -83.6781) knots 0 0 0 0 1 1 1 1
  line L377 (5.9357, -83.6781) -> (10.3552, -83.6781)
  line L378 (10.3552, -83.6781) -> (10.3552, -85.3635)
  line L379 (10.3552, -85.3635) -> (6.3516, -85.3635)
  spline S35 degree 3 poles (6.3516, -85.3635) (5.6413, -85.3635) (5.2864, -85.6005) (5.2864, -86.0711) knots 0 0 0 0 1 1 1 1
  spline S36 degree 3 poles (5.2864, -86.0711) (5.2864, -86.6051) (5.6642, -87.119) (6.4199, -87.613) knots 0 0 0 0 1 1 1 1
  line L380 (6.4199, -87.613) -> (10.3552, -87.613)
  line L381 (10.3552, -87.613) -> (10.3552, -89.2984)
  spline S37 degree 3 poles (10.321, -78.415) (10.4391, -78.8188) (10.4977, -79.1359) (10.4977, -79.3662) knots 0 0 0 0 1 1 1 1
  spline S38 degree 3 poles (10.4977, -79.3662) (10.4977, -80.828) (9.8143, -81.5589) (8.4474, -81.5589) knots 0 0 0 0 1 1 1 1
  line L382 (8.4474, -81.5589) -> (5.1556, -81.5589)
  line L383 (5.1556, -81.5589) -> (5.1556, -82.2597)
  line L384 (5.1556, -82.2597) -> (4.1016, -82.2597)
  line L385 (4.1016, -82.2597) -> (4.1016, -81.5589)
  line L386 (4.1016, -81.5589) -> (3.0481, -81.5589)
  line L387 (3.0481, -81.5589) -> (2.8543, -79.8735)
  line L388 (2.8543, -79.8735) -> (4.1016, -79.8735)
  line L389 (4.1016, -79.8735) -> (4.1016, -78.5352)
  line L390 (4.1016, -78.5352) -> (5.1556, -78.5352)
  line L391 (5.1556, -78.5352) -> (5.1556, -79.8735)
  line L392 (5.1556, -79.8735) -> (8.2252, -79.8735)
  spline S39 degree 3 poles (8.2252, -79.8735) (8.9922, -79.8735) (9.3759, -79.5598) (9.3759, -78.9323) knots 0 0 0 0 1 1 1 1
  spline S40 degree 3 poles (9.3759, -78.9323) (9.3759, -78.7888) (9.349, -78.6153) (9.2958, -78.415) knots 0 0 0 0 1 1 1 1
  line L393 (9.2958, -78.415) -> (10.321, -78.415)
extrude "Extrude5" add sketch "Sketch5" along normal blind 2 separate body contours L0 L1 L2 L3 makes body 2
named bodies: "Build Write Panel", "Count Panel"
